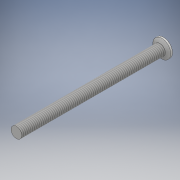
# Autodesk Inventor part: M3x40mm
Saved by Autodesk Inventor 2018 (Build 220112000, 112)
## iProperties
Created: 2017-11-05
Part Number: M3x40mm
Material: Generic
Document SubType Name: Modeling
Designer: Jurjen
Density: 1 g/cm^3
Appearance: Default
Author: Jurjen
Autodesk Inventor part; units mm, degrees
ref_plane "YZ Plane" through (0, 0, 0) normal (1, 0, 0) x (0, 1, 0)
ref_plane "XZ Plane" through (0, 0, 0) normal (0, 1, 0) x (-1, 0, 0)
ref_plane "XY Plane" through (0, 0, 0) normal (0, 0, 1) x (1, 0, 0)
sketch "Sketch1" plane through (0, 0, 0) normal (0, 0, 1) x (1, 0, 0)
  line L0 (0, -20.5) -> (1.5, -20.5)
  line L1 (1.5, -20.5) -> (1.5, 19.5)
  line L2 (2.5, 20.5) -> (0, 20.5)
  line L3 (0, 20.5) -> (0, -20.5)
  line L4 (1.5, 19.5) -> (2.5, 20)
  line L5 (2.5, 20) -> (2.5, 20.5)
  point P0 (0, 0)
  point P1 (0, 0)
  dimension "d0" = 1.5
  dimension "d1" = 41
  dimension "d2" = 2.5
  dimension "d3" = 40
  dimension "d15" = 0.5
  constraints: 12 end point, 2 perpendicular, 1 coincident, 1 horizontal, 1 midpoint, 1 parallel, 1 vertical, 1 vertical alignment
  measures "d0" distance between parallel lines of L3 L1
  measures "d1" distance of L2.end L0.start
  measures "d2" distance of L2.start L2.end
  measures "d3" distance of L0.end L1.end
  measures "d15" distance of L4.end L2.start
revolve "Revolution1" add sketch "Sketch1" angle 360 about axis through (0, 20.5, 0) along (0, -1, 0)
sketch "Sketch2" plane through (0, 20.5, 0) normal (0, 1, 0) x (1, 0, 0)
  line L0 (0, 1.2) -> (-0.4, 1.2)
  circle A0 centre (0, 0) radius 1.5 projected
  line L1 (-1.2, 0.4) -> (-1.2, 0)
  line L2 (-0.4, 1.2) -> (-0.4, 0.4)
  line L3 (-0.4, 0.4) -> (-1.2, 0.4)
  line L4 (-1.2, 0) -> (-1.2, -0.4)
  line L5 (-1.2, -0.4) -> (-0.4, -0.4)
  line L6 (-0.4, -0.4) -> (-0.4, -1.2)
  line L7 (-0.4, -1.2) -> (0, -1.2)
  line L8 (0, -1.2) -> (0.4, -1.2)
  line L9 (0.4, -1.2) -> (0.4, -0.4)
  line L10 (0.4, -0.4) -> (1.2, -0.4)
  line L11 (1.2, -0.4) -> (1.2, 0)
  line L12 (1.2, 0) -> (1.2, 0.4)
  line L13 (1.2, 0.4) -> (0.4, 0.4)
  line L14 (0.4, 0.4) -> (0.4, 1.2)
  line L15 (0.4, 1.2) -> (0, 1.2)
  line L16 (-1.2, -0.4) -> (-1.2, 0.4)
  line L17 (-0.4, 1.2) -> (0.4, 1.2)
  line L18 (1.2, -0.4) -> (1.2, 0.4)
  line L19 (0.4, -1.2) -> (-0.4, -1.2)
  point P0 (0, 0)
  dimension "d5" = 1.2
  dimension "d6" = 1.2
  dimension "d8" = 0.4
  dimension "d11" = 360
  constraints: 40 end point, 2 perpendicular, 2 vertical, 1 horizontal, 1 horizontal alignment, 1 vertical alignment, 37 other
  measures "d5" distance of point (0, 0) L1.end
  measures "d6" distance of point (0, 0) L0.start
  measures "d8" distance of L1.start L1.end
extrude "Extrusion1" cut sketch "Sketch2" against normal blind 0.5 contours L15 L14 L13 L12 L11 L10 L9 L8 L7 L6 L5 L4 L1 L3 L2 L0
thread "Thread1" size "M3x0.5" class "6g" standard "ANSI Metric M Profile" full length
chamfer "Chamfer1" distance 0.1 angle 45 12 edges at (-0.8, 20.5, -0.4) (-0.4, 20.5, -0.8) (0, 20.5, -1.2) (0.4, 20.5, -0.8) (0.8, 20.5, -0.4) (1.2, 20.5, 0) (0.8, 20.5, 0.4) (0.4, 20.5, 0.8) (0, 20.5, 1.2) (-0.4, 20.5, 0.8) (-1.2, 20.5, 0) (-0.8, 20.5, 0.4)
equation "\"d6\" = d5"
body "Solid1"
